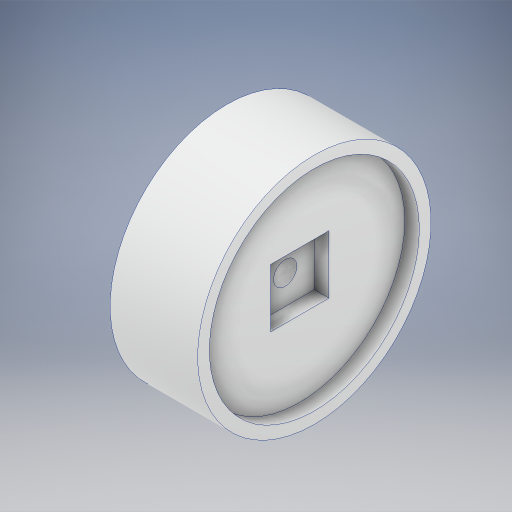
# Autodesk Inventor part: wheel
Saved by Autodesk Inventor 2024 (Build 280153000, 153)
## iProperties
Created: 2024-04-09
Part Number: wheel
Material: Aluminum 6061
Document SubType Name: Modeling
Designer: Alex
Density: 2.7 g/cm^3
Appearance: Aluminum - Flat
Mass: 199.023 g
Surface Area: 247.411 cm^2
Volume: 73.7124 cm^3
Author: Alex
Autodesk Inventor part; units mm, degrees
sketch "Sketch3" plane through (0, 0, 0) normal (1, 0, 0) x (0, 1, 0)
  circle A0 centre (0, 0) radius 40
  circle A1 centre (0, 0) radius 5
  dimension "d2" = 80
  dimension "d3" = 10
  constraints: 2 centre point, 2 coincident
  measures "d2" diameter of A0
  measures "d3" diameter of A1
extrude "Extrusion1" add sketch "Sketch3" along normal blind 30 contours A0 | A1
sketch "Sketch4" plane through (30, 0, 0) normal (1, 0, 0) x (0, 0, -1)
  circle A0 centre (0, 0) radius 5 construction
  circle A1 centre (0, 0) radius 36
  circle A2 centre (0, 0) radius 40 projected
  dimension "d6" = 4
  constraints: 2 centre point, 2 coincident
  measures "d6" radial gap between concentric circles of A1 A2
ref_plane "Work Plane1" through (15, 0, 0) normal (-1, 0, 0) x (0, 0, 1)
extrude "Extrusion2" cut sketch "Sketch4" against normal blind 10 contours A1
sketch "Sketch5" plane through (20, 0, 0) normal (1, 0, 0) x (0, 0, -1)
  circle A0 centre (0, 0) radius 4
  circle A1 centre (0, 0) radius 36 construction
  dimension "d12" = 8
  constraints: 1 centre point, 1 coincident
  measures "d12" diameter of A0
extrude "Extrusion3" cut sketch "Sketch5" against normal up to next
sketch "Sketch6" plane through (20, 0, 0) normal (1, 0, 0) x (0, 0, -1)
  circle A0 centre (0, 0) radius 4 projected
  circle A1 centre (0, 0) radius 36 projected
  line L0 (-10, 10) -> (10, 10)
  line L1 (10, 10) -> (10, -10)
  line L2 (10, -10) -> (-10, -10)
  line L3 (-10, -10) -> (-10, 10)
  line L4 (-10, 10) -> (10, -10) construction
  line L5 (10, 10) -> (-10, -10) construction
  dimension "d13" = 20
  constraints: 12 end point, 2 midpoint, 2 parallel, 2 perpendicular, 1 horizontal
  measures "d13" distance of L1.end L2.end
extrude "Extrusion4" add sketch "Sketch6" along normal up to surface (10 mm away) contours A1
ref_plane "Work Plane2" through (15, 0, 0) normal (1, 0, 0) x (0, 0, -1)
sketch "Sketch7" plane through (30, 0, 0) normal (1, 0, 0) x (0, 0, -1)
  circle A0 centre (0, 0) radius 36 projected
extrude "Extrusion5" cut sketch "Sketch7" against normal blind 5
sketch "Sketch8" plane through (0, 0, 0) normal (-1, 0, 0) x (0, 0, 1)
  circle A0 centre (0, 0) radius 36 projected
  circle A1 centre (0, 0) radius 4 projected
extrude "Extrusion6" cut sketch "Sketch8" against normal blind 15
sketch "Sketch9" plane through (15, 0, 0) normal (-1, 0, 0) x (0, 0, 1)
  circle A0 centre (0, 0) radius 4 projected
  circle A1 centre (0, 0) radius 10
  dimension "d21" = 20
  constraints: 1 centre point, 1 coincident
  measures "d21" diameter of A1
extrude "Extrusion7" add sketch "Sketch9" along normal blind 25
sketch "Sketch10" plane through (15, 0, 0) normal (-1, 0, 0) x (0, 0, 1)
  line L0 (0, 0) -> (28.2843, 28.2843)
  line L1 (0, 0) -> (-28.2843, 28.2843)
  circle A0 centre (0, 0) radius 40 projected
  circle A1 centre (0, 0) radius 4 construction
  line L2 (0, 0) -> (0, 40) construction
  dimension "d24" = 90
  constraints: 6 end point, 3 point on circle, 1 vertical, 1 other
  measures "d24" angle of L1 L0
ref_plane "Work Plane3" through (0, 40, 0) normal (0, 1, 0) x (-1, 0, 0)
body "Solid1"
